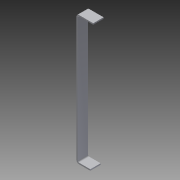
# Autodesk Inventor part: LANcrossmember
Saved by Autodesk Inventor 2014 (Build 180170000, 170)
## iProperties
Created: 2013-10-21
Part Number: LANcrossmember
Material: Aluminum 6061
Document SubType Name: Sheet Metal
Designer: 14hensgenw
Density: 2.71 g/cm^3
Sheet Metal Rule: Default
Appearance: Aluminum - Flat
Author: 14hensgenw
Autodesk Inventor part; units mm, degrees
ref_plane "YZ Plane" through (0, 0, 0) normal (1, 0, 0) x (0, 1, 0)
ref_plane "XZ Plane" through (0, 0, 0) normal (0, 1, 0) x (-1, 0, 0)
ref_plane "XY Plane" through (0, 0, 0) normal (0, 0, 1) x (1, 0, 0)
sketch "Sketch1" plane through (0, 0, 0) normal (0, 1, 0) x (-1, 0, 0)
  line L0 (206.402, -59.3979) -> (-174.598, -59.3979)
  line L1 (-174.598, -59.3979) -> (-174.598, -33.9979)
  line L2 (-174.598, -33.9979) -> (206.402, -33.9979)
  line L3 (206.402, -33.9979) -> (206.402, -59.3979)
  point P0 (0, 0)
  dimension "d0" = 381
  dimension "d1" = 25.4
  measures "d0" distance of L0.start L0.end
  measures "d1" distance of L2.end L0.start
extrude "Plate1" add sketch "Sketch1" along normal blind 3.175
sketch "Sketch2" plane through (0, 3.175, 0) normal (0, 1, 0) x (1, 0, 0)
  line L0 (-206.402, 59.3979) -> (174.598, 59.3979) projected
  line L1 (174.598, 33.9979) -> (-206.402, 33.9979) projected
  line L2 (-15.902, 33.9979) -> (139.673, 33.9979)
  line L3 (-15.902, 33.9979) -> (-171.477, 33.9979)
  line L4 (-171.477, 33.9979) -> (-171.477, 59.3979)
  line L5 (139.673, 33.9979) -> (139.673, 59.3979)
  point P0 (0, 0)
  dimension "d4" = 155.575
  dimension "d5" = 155.575
  constraints: 8 end point, 4 point on line, 2 perpendicular, 1 midpoint
  measures "d4" distance of L2.start L2.end
  measures "d5" distance of L2.start L3.end
fold "Fold1" angle 90 bend radius 3.175 thickness 3.175 k factor 0.44 line from (-171.477, 3.175, -33.9979) to (-171.477, 3.175, -59.3979) line at bend end moving side (-1, 0, 0) folds toward (0, 1, 0)
fold "Fold2" angle 90 bend radius 3.175 thickness 3.175 k factor 0.44 line from (139.673, 3.175, -33.9979) to (139.673, 3.175, -59.3979) line at bend end moving side (-1, 0, 0) folds toward (0, 1, 0)
sketch "Sketch3" plane through (146.8547, 316.6683, -33.9979) normal (0, 1, 0) x (1, 0, 0)
  line L0 (0, 25.4) -> (0, 0) projected
  line L1 (0, 0) -> (34.925, 0) projected
  line L2 (34.925, 0) -> (34.925, 25.4) projected
  line L3 (34.925, 25.4) -> (0, 25.4) projected
  point P0 (-146.8547, -33.9979)
equation "\"d6\" = BendReliefWidth"
equation "\"d7\" = BendReliefDepth"
equation "\"d8\" = MinimumRemnant"
equation "\"d9\" = BendRadius"
equation "\"d11\" = BendRadius"
equation "\"d12\" = BendReliefWidth"
equation "\"d13\" = BendReliefDepth"
equation "\"d14\" = MinimumRemnant"
equation "\"d15\" = BendRadius"
equation "\"d17\" = BendRadius"
equation "\"BendRadius\" = Thickness"
equation "\"BendReliefWidth\" = Thickness"
equation "\"BendReliefDepth\" = 0.5 * Thickness"
equation "\"CornerReliefSize\" = 4 * Thickness"
equation "\"MinimumRemnant\" = 2 * Thickness"
equation "\"TransitionRadius\" = BendRadius"
equation "\"JacobiRadiusSize\" = Thickness"
equation "\"GapSize\" = Thickness"
equation "\"d2\" = BendRadius"
equation "\"Thickness\" = 3.175"
body "Solid1"
